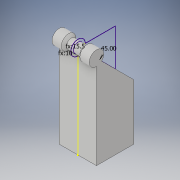
# Autodesk Inventor part: upper leg V2
Saved by Autodesk Inventor 2019 (Build 230136000, 136)
## iProperties
Created: 2018-07-06
Part Number: upper leg V2
Material: Generic
Document SubType Name: Modeling
Designer: HIVE
Density: 1 g/cm^3
Appearance: Default
Author: HIVE
Autodesk Inventor part; units mm, degrees
ref_plane "YZ Plane" through (0, 0, 0) normal (1, 0, 0) x (0, 1, 0)
ref_plane "XZ Plane" through (0, 0, 0) normal (0, 1, 0) x (-1, 0, 0)
ref_plane "XY Plane" through (0, 0, 0) normal (0, 0, 1) x (1, 0, 0)
sketch "Sketch1" plane through (0, 0, 0) normal (0, 1, 0) x (-1, 0, 0)
  line L0 (0, 0) -> (40, 0)
  line L1 (40, 0) -> (40, -40)
  line L2 (40, -40) -> (0, -40)
  line L3 (0, -40) -> (0, 0)
  dimension "d2" = 40
  dimension "d3" = 40
  constraints: 8 end point, 2 parallel, 1 horizontal, 1 perpendicular
  measures "d2" distance of L1.end L2.end
  measures "d3" distance of L0.end L1.end
extrude "Extrusion1" add sketch "Sketch1" along normal blind 100
ref_plane "Work Plane1" through (-20, 0, 0) normal (1, 0, 0) x (0, 0, -1)
sketch "Sketch2" plane through (-20, 0, 0) normal (1, 0, 0) x (0, 0, -1)
  line L0 (40, 0) -> (0, 0) projected
  line L1 (40, 0) -> (40, 100) projected
  line L2 (0, 100) -> (40, 100) projected
  line L3 (0, 0) -> (0, 100) projected
  circle A0 centre (0, 100) radius 5
  line L4 (40, 100) -> (0, 100) projected
  arc A1 (7.75, 100) -> (5.4801, 94.5199) centre (0, 100) ccw
  line L5 (5.4801, 94.5199) -> (40, 60)
  line L6 (40, 0) -> (40, 100) projected
  line L7 (40, 100) -> (40, 60)
  line L8 (40, 100) -> (7.75, 100)
  arc A2 (5.4801, 94.5199) -> (7.75, 100) centre (0, 100) ccw
  dimension "d4" = 15.5
  dimension "d5" = 10
  dimension "d16" = 45
  constraints: 6 end point, 4 point on circle, 3 centre point, 3 point on line, 2 coincident, 1 collinear
  measures "d4" diameter of A1
  measures "d5" diameter of A0
  measures "d16" angle of L1 L5
extrude "Extrusion2" add sketch "Sketch2" along normal mid plane 40 contours A1 L2 A0 L3 | L3 A0 L2 A2 A1
extrude "Extrusion3" cut sketch "Sketch2" along normal mid plane 40 contours A0 L2 L3 | L3 L2 A0
extrude "Extrusion4" cut sketch "Sketch2" along normal mid plane 20 contours A1 L2 A0 L3 | L3 A0 L2 A2 A1
extrude "Extrusion6" cut sketch "Sketch2" along normal mid plane 40 contours L5 A2 L2 L1
extrude "Extrusion7" add sketch "Sketch2" along normal mid plane 40 contours A0 L2 L3 | L3 L2 A0
chamfer "Chamfer1" distance 2.75 angle 45 1 edges at (-30, 100, 5) measured on face at (-30, 100, 5.5)
chamfer "Chamfer2" distance 2.75 angle 45 1 edges at (-10, 100, 5) measured on face at (-10, 100, 5.5)
equation "\"d2\" = legDiam"
equation "\"d3\" = legDiam"
equation "\"d5\" = hingeHoleDiam"
equation "\"d6\" = legDiam"
equation "\"d8\" = legDiam"
equation "\"d10\" = 0.5 * legDiam"
equation "\"d17\" = legDiam"
equation "\"d19\" = legDiam"
equation "\"d21\" = -0.5 * d5 + 0.5 * d4"
equation "\"d24\" = -0.5 * d5 + 0.5 * d4"
equation "\"legDiam\" = 40"
equation "\"hingeHoleDiam\" = 10"
body "Solid1"
